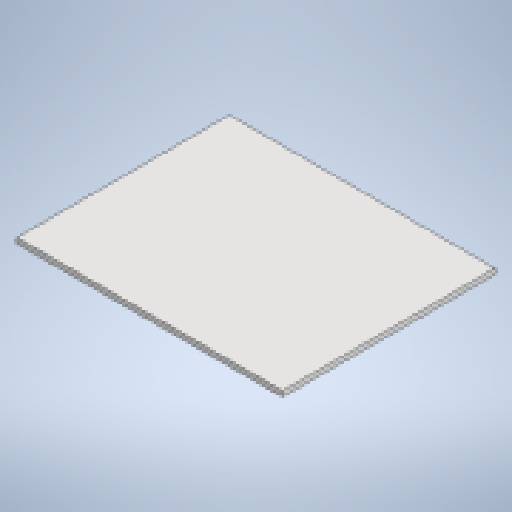
# Autodesk Inventor part: roof
Saved by Autodesk Inventor 2023 (Build 270158000, 158)
## iProperties
Created: 2022-10-04
Part Number: roof
Material: Generic
Document SubType Name: Modeling
Designer: carso
Density: 1 g/cm^3
Appearance: Default
Author: carso
Autodesk Inventor part; units mm, degrees
ref_plane "YZ Plane" through (0, 0, 0) normal (1, 0, 0) x (0, 1, 0)
ref_plane "XZ Plane" through (0, 0, 0) normal (0, 1, 0) x (-1, 0, 0)
ref_plane "XY Plane" through (0, 0, 0) normal (0, 0, 1) x (1, 0, 0)
sketch "Sketch1" plane through (0, 0, 0) normal (0, 1, 0) x (-1, 0, 0)
  line L0 (88.6302, -47.0481) -> (-111.3698, -47.0481)
  line L1 (-111.3698, -47.0481) -> (-111.3698, 112.9519)
  line L2 (-111.3698, 112.9519) -> (88.6302, 112.9519)
  line L3 (88.6302, 112.9519) -> (88.6302, -47.0481)
  point P0 (0, 0)
  dimension "d0" = 200
  dimension "d1" = 160
  constraints: 8 end point, 2 parallel, 1 horizontal, 1 perpendicular
  measures "d0" distance of L0.start L0.end
  measures "d1" distance of L2.end L0.start
extrude "Extrusion1" add sketch "Sketch1" along normal blind 4
sketch "Sketch3" plane through (0, 0, 0) normal (0, -1, 0) x (1, 0, 0)
  line L0 (111.3698, 112.9519) -> (111.3698, -47.0481) projected
  line L1 (111.3698, 32.9519) -> (-88.6302, 32.9519)
  line L2 (-88.6302, -47.0481) -> (-88.6302, 112.9519) projected
  point P0 (0, 0)
  constraints: 2 end point, 2 midpoint
body "Solid1"
